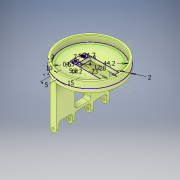
# Autodesk Inventor part: Mouth-Base
Saved by Autodesk Inventor 2018.3 (Build 223284000, 284)
## iProperties
Created: 2018-05-16
Part Number: Mouth-Base
Material: Generisch
Document SubType Name: Modeling
Designer: JochenAlt
Density: 1 g/cm^3
Appearance: Vorgabe
Author: JochenAlt
Autodesk Inventor part; units mm, degrees
ref_plane "YZ Plane" through (0, 0, 0) normal (1, 0, 0) x (0, 1, 0)
ref_plane "XZ Plane" through (0, 0, 0) normal (0, 1, 0) x (-1, 0, 0)
ref_plane "XY Plane" through (0, 0, 0) normal (0, 0, 1) x (1, 0, 0)
sketch "Skizze1" plane through (0, 0, 0) normal (0, 0, 1) x (1, 0, 0)
  circle A0 centre (0, 0) radius 22.1
  line L0 (0, 33.74) -> (0, -33.74) construction
  line L1 (-33.74, 0) -> (33.74, 0) construction
  circle A1 centre (0, 0) radius 24.1
  line L2 (-5.8, -6) -> (17.2, -6)
  line L3 (17.2, -6) -> (17.2, 6)
  line L4 (17.2, 6) -> (-5.8, 6)
  line L5 (-5.8, 6) -> (-5.8, -6)
  line L6 (-5.8, -6) -> (-10.3, -6)
  line L7 (-10.3, -6) -> (-10.3, 6)
  line L8 (-10.3, 6) -> (-5.8, 6)
  line L9 (-8.3, -3.5) -> (-8.3, 3.5) construction
  circle A2 centre (-8.3, -3.5) radius 0.85
  circle A3 centre (-8.3, 3.5) radius 0.85
  line L10 (17.2, -6) -> (21.7, -6)
  line L11 (21.7, -6) -> (21.7, 6)
  line L12 (21.7, 6) -> (17.2, 6)
  line L13 (19.7, -3.5) -> (19.7, 3.5) construction
  circle A4 centre (19.7, -3.5) radius 0.85
  circle A5 centre (19.7, 3.5) radius 0.85
  line L14 (5.7, -6) -> (5.7, 6) construction
  circle A6 centre (-8.3, 3.5) radius 2
  circle A7 centre (-8.3, -3.5) radius 2
  circle A8 centre (19.7, 3.5) radius 2
  circle A9 centre (19.7, -3.5) radius 2
  arc A10 (19.1836, 6) -> (19.1836, -6) centre (0, 0) ccw
  dimension "d0" = 44.2
  dimension "d2" = 2
  dimension "d11" = 5.8
  dimension "d12" = 23
  dimension "d13" = 12
  dimension "d14" = 4.5
  dimension "d16" = 7
  dimension "d21" = 28
  dimension "d22" = 1.7
  dimension "d23" = 4
  constraints: 26 end point, 11 centre point, 10 coincident, 6 equal radius, 5 perpendicular, 3 horizontal, 2 midpoint, 2 parallel, 2 point on circle, 2 point on line, 2 vertical, 1 collinear, 1 symmetric about line, 2 other
  measures "d0" diameter of A0
  measures "d2" radial gap between concentric circles of A1 A0
  measures "d11" distance between parallel lines of L0 L5
  measures "d12" distance between parallel lines of L3 L5
  measures "d13" distance between parallel lines of L4 L2
  measures "d14" distance between parallel lines of L5 L7
  measures "d16" distance of L9.start L9.end
  measures "d21" distance between parallel lines of L13 L9
  measures "d22" diameter of A3
  measures "d23" diameter of A6
extrude "Extrusion1" add sketch "Skizze1" along normal blind 5 contours A0 L12 L11 | L11 L10 A0 | A1
extrude "Extrusion2" add sketch "Skizze1" against normal blind 3 contours A0 L11 | A9 | A8 | L11 A0 L10 L3 L12 | A0 L12 L11 | L11 L10 A0 | L12 A10 L10 A0 | L12 L4 L8 L7 L6 L2 L10 A10 | A6 | A7 | L5 L6 L7 L8 | A1
chamfer "Fase1" distance 0.5 angle 45 1 edges at (-22.1, 0, 5)
extrude "Extrusion3" add sketch "Skizze1" against normal blind 2 from surface at -3 contours A9 | A8 | L11 A0 L10 L3 L12 | A0 L12 L11 | L11 L10 A0 | A6 | A7 | L5 L6 L7 L8
extrude "Extrusion4" cut sketch "Skizze1" against normal blind 2 contours A9 | A8 | A6 | A7 | A2 | A3 | A4 | A5
sketch "Skizze3" plane through (0, 0, -3) normal (0, 0, -1) x (-1, 0, 0)
  line L0 (0, -33.74) -> (0, 33.74) construction
  line L1 (-33.74, 0) -> (33.74, 0) construction
  line L2 (10.8, -21.5) -> (5.8, -21.5)
  line L3 (5.8, -21.5) -> (5.8, -6.5)
  line L4 (5.8, -6.5) -> (10.8, -6.5)
  line L5 (10.8, -6.5) -> (10.8, -21.5)
  line L6 (10.8, 6.5) -> (5.8, 6.5)
  line L7 (5.8, 6.5) -> (5.8, 21.5)
  line L8 (5.8, 21.5) -> (10.8, 21.5)
  line L9 (10.8, 21.5) -> (10.8, 6.5)
  line L10 (10.8, -19.5) -> (5.8, -19.5)
  line L11 (10.8, -8.5) -> (5.8, -8.5)
  line L12 (10.8, 8.5) -> (5.8, 8.5)
  line L13 (10.8, 19.5) -> (5.8, 19.5)
  line L14 (5.8, -6) -> (-17.2, -6) projected
  line L15 (10.8, -6.5) -> (10.8, 6.5)
  line L16 (5.8, -6.5) -> (5.8, 6.5)
  line L17 (20.8, -8.5) -> (10.8, -8.5)
  line L18 (10.8, -6.5) -> (20.8, -6.5)
  line L19 (20.8, -6.5) -> (20.8, -8.5)
  line L20 (20.8, 6.5) -> (10.8, 6.5)
  line L21 (10.8, 8.5) -> (20.8, 8.5)
  line L22 (20.8, 8.5) -> (20.8, 6.5)
  line L23 (5.8, 6) -> (5.8, -6) projected
  point P0 (0, 0)
  dimension "d26" = 5
  dimension "d27" = 15
  dimension "d29" = 2
  dimension "d30" = 2
  dimension "d36" = 0.5
  dimension "d46" = 2
  dimension "d55" = 10
  constraints: 40 end point, 12 point on line, 7 horizontal, 6 parallel, 4 collinear, 4 perpendicular, 2 equal length, 5 other
  measures "d26" distance of L2.start L2.end
  measures "d27" distance of L2.end L3.end
  measures "d29" distance between parallel lines of L10 L2
  measures "d30" distance between parallel lines of L4 L11
  measures "d36" distance between parallel lines of L14 L4
  measures "d46" distance of L18.end L17.start
  measures "d55" distance of L17.start L17.end
extrude "Extrusion5" add sketch "Skizze3" along normal blind 30 contours L2 L3 L10 L5 | L10 L3 L11 L5 | L11 L3 L4 L5 | L6 L7 L12 L9 | L12 L7 L13 L9 | L13 L7 L8 L9
extrude "Extrusion6" add sketch "Skizze3" along normal blind 8 from surface at 30 contours L2 L3 L10 L5 | L11 L3 L4 L5 | L6 L7 L12 L9 | L13 L7 L8 L9
fillet "Rundung1" radius 2.5 8 edges at (-10.8, -7.5, -41) (-5.8, -7.5, -41) (-10.8, -20.5, -41) (-5.8, -20.5, -41) (-10.8, 7.5, -41) (-5.8, 7.5, -41) (-10.8, 20.5, -41) (-5.8, 20.5, -41)
extrude "Extrusion7" add sketch "Skizze3" against normal blind 2 from surface at 30 contours L4 L16 L6 L15
sketch "Skizze4" plane through (-10.8, 21.5, -3) normal (0, 1, 0) x (1, 0, 0)
  arc A0 (5, 35.5) -> (0, 35.5) centre (2.5, 35.5) ccw projected
  circle A1 centre (2.5, 35.5) radius 1
  point P0 (10.8, -3)
  dimension "d41" = 2
  constraints: 2 coincident, 1 centre point
  measures "d41" diameter of A1
extrude "Extrusion8" cut sketch "Skizze4" against normal through all
fillet "Rundung2" radius 2 8 edges at (-8.3, -19.5, -33) (-8.3, -8.5, -33) (-8.3, 19.5, -33) (-8.3, 8.5, -33) (-8.3, -6.5, -31) (-8.3, 6.5, -31) (-8.3, -6.5, -33) (-8.3, 6.5, -33)
extrude "Extrusion9" add sketch "Skizze3" along normal up to surface (30 mm away) contours L5 L18 L19 L17 | L9 L21 L22 L20
chamfer "Fase2" distance 30 distance2 10 1 edges at (-20.8, -7.5, -33) measured on face at (-20.8, -7.5, -32.5)
chamfer "Fase3" distance 30 distance2 10 1 edges at (-20.8, 7.5, -33) measured on face at (-20.8, 7.5, -32.5)
equation "\"d30\" = d29"
equation "\"d35\" = 0.5 * d26"
